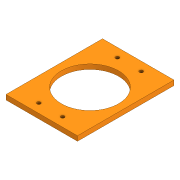
# Autodesk Inventor part: payload-plateV2
Saved by Autodesk Inventor 2020.3 (Build 243373000, 373)
## iProperties
Created: 2021-06-12
Part Number: payload-plateV2
Material: Generic
Document SubType Name: Modeling
Designer: Yusuf
Mass: 12.0887 g
Surface Area: 79.2632 cm^2
Volume: 12.0887 cm^3
Density: 1 g/cm^3
Appearance: Orange
Author: Yusuf
Autodesk Inventor part; units mm, degrees
ref_plane "YZ Plane" through (0, 0, 0) normal (1, 0, 0) x (0, 1, 0)
ref_plane "XZ Plane" through (0, 0, 0) normal (0, 1, 0) x (-1, 0, 0)
ref_plane "XY Plane" through (0, 0, 0) normal (0, 0, 1) x (1, 0, 0)
sketch "Sketch1" plane through (0, 0, 0) normal (0, 1, 0) x (-1, 0, 0)
  line L0 (0, 0) -> (60, 0)
  line L1 (60, 0) -> (60, -81)
  line L2 (60, -81) -> (0, -81)
  line L3 (0, -81) -> (0, 0)
  line L4 (45, -21.6284) -> (15, -21.6284) construction
  line L5 (45, -81) -> (45, 0) construction
  line L6 (15, 0) -> (15, -81) construction
  circle A0 centre (40, -73.5) radius 1.5
  circle A1 centre (40, -7.5) radius 1.5
  circle A2 centre (20, -7.5) radius 1.5
  circle A3 centre (20, -73.5) radius 1.5
  circle A4 centre (30, -40.5) radius 24
  point P0 (30, -21.6284)
  point P1 (30, -81)
  dimension "width" = 60
  dimension "d1" = 81
  dimension "fixed" = 3
  dimension "d6" = 7.5
  dimension "d7" = 5
  dimension "d8" = 30
  dimension "d9" = 3
  dimension "d10" = 7.5
  dimension "d11" = 5
  dimension "d12" = 3
  dimension "d13" = 3
  dimension "d14" = 5
  dimension "d15" = 48
  constraints: 14 end point, 6 point on line, 5 centre point, 3 perpendicular, 2 horizontal, 2 horizontal alignment, 2 midpoint, 2 parallel, 2 vertical alignment
  measures "width" distance of L1.end L2.end
  measures "d1" distance of L0.end L1.end
  measures "fixed" diameter of A0
  measures "d6" distance from line of A0.centre L2
  measures "d7" distance from line of L5 A0.centre
  measures "d8" distance between parallel lines of L6 L5
  measures "d9" diameter of A1
  measures "d10" distance from line of L0 A1.centre
  measures "d11" distance from line of L5 A1.centre
  measures "d12" diameter of A2
  measures "d13" diameter of A3
  measures "d14" distance from line of L6 A2.centre
  measures "d15" diameter of A4
extrude "Extrusion1" add sketch "Sketch1" along normal blind 4
equation "\"d8\" = 0.5 * width"
equation "\"d9\" = fixed"
equation "\"d12\" = fixed"
equation "\"d13\" = fixed"
body "Solid1"
